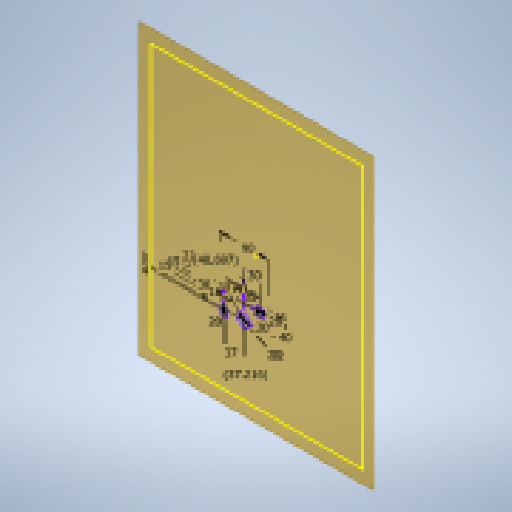
# Autodesk Inventor part: mode-control-layout
Saved by Autodesk Inventor 2023 (Build 270158030, 158C)
## iProperties
Created: 2024-04-02
Part Number: mode-control-layout
Material: Generic
Document SubType Name: Modeling
Designer: Imogen Heard
Density: 1 g/cm^3
Appearance: Default
Author: Imogen Heard
Autodesk Inventor part; units mm, degrees
ref_plane "YZ Plane" through (0, 0, 0) normal (1, 0, 0) x (0, 1, 0)
ref_plane "XZ Plane" through (0, 0, 0) normal (0, 1, 0) x (-1, 0, 0)
ref_plane "XY Plane" through (0, 0, 0) normal (0, 0, 1) x (1, 0, 0)
ref_plane "Work Plane1" through (0, 0, 0) normal (0, 0, 1) x (1, 0, 0)
sketch "Sketch1" plane through (0, 0, 0) normal (0, 0, 1) x (1, 0, 0)
  line L0 (-68.1954, -80.0527) -> (21.8046, -80.0527) construction
  line L1 (21.8046, -80.0527) -> (21.8046, -58.0527) construction
  line L2 (21.8046, -58.0527) -> (-68.1954, -58.0527) construction
  line L3 (-68.1954, -58.0527) -> (-68.1954, -80.0527) construction
  circle A0 centre (-23.1954, -120.0527) radius 11
  line L4 (-19.6974, 112.8804) -> (-26.8098, -352.984) construction
  line L5 (-26.8098, -352.984) -> (-26.7516, -352.9849) construction
  line L6 (-26.7516, -352.9849) -> (-19.6392, 112.8795) construction
  line L7 (-19.6392, 112.8795) -> (-19.6974, 112.8804) construction
  line L8 (-40.6954, -100.0527) -> (-5.6954, -100.0527) construction
  line L9 (-5.6954, -100.0527) -> (-5.6954, -90.0527) construction
  line L10 (-5.6954, -90.0527) -> (-40.6954, -90.0527) construction
  line L11 (-40.6954, -90.0527) -> (-40.6954, -100.0527) construction
  line L12 (-75.1954, -94.0527) -> (-75.1954, -104.0527) construction
  line L13 (-75.1954, -104.0527) -> (-45.1954, -104.0527) construction
  line L14 (-45.1954, -104.0527) -> (-45.1954, -94.0527) construction
  line L15 (-45.1954, -94.0527) -> (-75.1954, -94.0527) construction
  circle A1 centre (-23.1954, -120.0527) radius 14.5 construction
  circle A2 centre (6.8046, -95.0527) radius 8
  circle A3 centre (-60.1954, -124.0527) radius 8
  circle A4 centre (6.8046, -95.0527) radius 10 construction
  circle A5 centre (-60.1954, -124.0527) radius 10 construction
  line L16 (-198, -244.5) -> (198, -244.5) projected
  line L17 (198, -244.5) -> (198, 244.5) projected
  line L18 (198, 244.5) -> (-198, 244.5) projected
  line L19 (-198, 244.5) -> (-198, -244.5) projected
  line L20 (-75.1954, -94.0527) -> (-45.1954, -94.0527)
  line L21 (-45.1954, -94.0527) -> (-45.1954, -104.0527)
  line L22 (-45.1954, -104.0527) -> (-75.1954, -104.0527)
  line L23 (-75.1954, -104.0527) -> (-75.1954, -94.0527)
  line L24 (-40.6954, -90.0527) -> (-5.6954, -90.0527)
  line L25 (-5.6954, -90.0527) -> (-5.6954, -100.0527)
  line L26 (-5.6954, -100.0527) -> (-40.6954, -100.0527)
  line L27 (-40.6954, -100.0527) -> (-40.6954, -90.0527)
  line L28 (-58.1954, -62.8527) -> (11.8046, -62.8527)
  line L29 (11.8046, -62.8527) -> (11.8046, -75.7527)
  line L30 (11.8046, -75.7527) -> (-58.1954, -75.7527)
  line L31 (-58.1954, -75.7527) -> (-58.1954, -62.8527)
  point P0 (0, 0)
  point P1 (-23.1954, -80.0527)
  point P2 (-23.1954, -100.0527)
  point P3 (-60.1954, -94.0527)
  point P4 (-60.1954, -104.0527)
  point P5 (-5.6954, -95.0527)
  point P6 (-23.1954, -90.0527)
  point P7 (-23.1954, -58.0527)
  dimension "d0" = 22
  dimension "d1" = 22
  dimension "d2" = 90
  dimension "d7" = 29
  dimension "d8" = 16
  dimension "d9" = 16
  dimension "d10" = 20
  dimension "d11" = 20
  dimension "d12" = 30
  dimension "d13" = 30
  dimension "d14" = 40
  dimension "d17" = 37
  dimension "d18" = 20
  dimension "d19" = 10
  dimension "d20" = 10
  dimension "d21" = 30
  dimension "d22" = 35
  dimension "d23" = 4
  dimension "d26" = 39.0513
  dimension "d27" = 37.2156
  dimension "d28" = 4.3
  dimension "d29" = 4.8
  dimension "d30" = 10
  dimension "d31" = 10
  constraints: 24 end point, 8 midpoint, 6 centre point, 6 parallel, 6 vertical alignment, 4 coincident, 3 horizontal, 3 perpendicular, 1 horizontal alignment, 8 other
  measures "d0" diameter of A0
  measures "d1" distance between parallel lines of L0 L2
  measures "d2" distance between parallel lines of L1 L3
  measures "d7" diameter of A1
  measures "d8" diameter of A2
  measures "d9" diameter of A3
  measures "d10" diameter of A4
  measures "d11" diameter of A5
  measures "d12" horizontal distance of A2.centre point (-23.195, -100.053)
  measures "d13" distance of point (-60.195, -94.053) A3.centre
  measures "d14" distance from line of A0.centre L0
  measures "d17" horizontal distance of A3.centre A0.centre
  measures "d18" distance from line of A0.centre L8
  measures "d19" distance between parallel lines of L8 L10
  measures "d20" distance between parallel lines of L13 L15
  measures "d21" distance between parallel lines of L14 L12
  measures "d22" distance between parallel lines of L9 L11
  measures "d23" vertical distance of A3.centre A0.centre
  measures "d26" distance of A0.centre A4.centre
  measures "d27" distance of A3.centre A0.centre
  measures "d28" distance between parallel lines of L0 L30
  measures "d29" distance between parallel lines of L2 L28
  measures "d30" distance between parallel lines of L1 L29
  measures "d31" distance between parallel lines of L3 L31
extrude "Extrusion1" add sketch "Sketch1" along normal blind 1 contours A0 | A2 | A3 | L20 L21 L22 L23 | L24 L25 L26 L27 | L28 L29 L30 L31
sketch "Sketch5" plane through (0, 0, 1) normal (0, 0, 1) x (1, 0, 0)
  line L0 (-55.571, -65.5595) -> (9.6532, -65.5595) construction
  line L1 (9.6532, -65.5595) -> (9.6532, -73.7983) construction
  line L2 (9.6532, -73.7983) -> (-55.571, -73.7983) construction
  line L3 (-55.571, -73.7983) -> (-55.571, -65.5595) construction
  point P0 (0, 0)
  constraints: 1 horizontal, 2 other
decal "Decal1"
sketch "Sketch6" plane through (0, 0, 1) normal (0, 0, 1) x (1, 0, 0)
  line L0 (-74.0258, -95.5765) -> (-46.8021, -95.5765) construction
  line L1 (-46.8021, -95.5765) -> (-46.8021, -102.7354) construction
  line L2 (-46.8021, -102.7354) -> (-74.0258, -102.7354) construction
  line L3 (-74.0258, -102.7354) -> (-74.0258, -95.5765) construction
  point P0 (0, 0)
  constraints: 1 horizontal, 2 other
decal "Decal2"
sketch "Sketch7" plane through (0, 0, 1) normal (0, 0, 1) x (1, 0, 0)
  line L0 (-38.5335, -91.962) -> (-7.4329, -91.962) construction
  line L1 (-7.4329, -91.962) -> (-7.4329, -98.548) construction
  line L2 (-7.4329, -98.548) -> (-38.5335, -98.548) construction
  line L3 (-38.5335, -98.548) -> (-38.5335, -91.962) construction
  point P0 (0, 0)
  constraints: 2 other
decal "Decal3"
